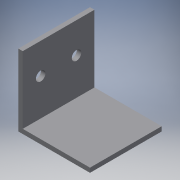
# Autodesk Inventor part: rail gusset
Saved by Autodesk Inventor 2016 (Build 200138000, 138)
## iProperties
Created: 2016-02-08
Part Number: rail gusset
Material: Generic
Document SubType Name: Modeling
Designer: gus
Density: 1 g/cm^3
Appearance: Default
Author: gus
Autodesk Inventor part; units mm, degrees
ref_plane "YZ Plane" through (0, 0, 0) normal (1, 0, 0) x (0, 1, 0)
ref_plane "XZ Plane" through (0, 0, 0) normal (0, 1, 0) x (-1, 0, 0)
ref_plane "XY Plane" through (0, 0, 0) normal (0, 0, 1) x (1, 0, 0)
sketch "Sketch1" plane through (0, 0, 0) normal (0, 0, 1) x (1, 0, 0)
  line L0 (0, 0) -> (47.625, 0)
  line L1 (47.625, 0) -> (47.625, -3.175)
  line L2 (47.625, -3.175) -> (-3.175, -3.175)
  line L3 (-3.175, -3.175) -> (-3.175, 47.625)
  line L4 (-3.175, 47.625) -> (0, 47.625)
  line L5 (0, 47.625) -> (0, 0)
  dimension "d14" = 50.8
  dimension "d15" = 3.175
  constraints: 12 end point, 6 perpendicular, 1 parallel, 1 vertical
  measures "d14" distance of L1.end L2.end
  measures "d15" distance of L0.end L1.end
extrude "Extrusion1" add sketch "Sketch1" along normal blind 50.8
sketch "Sketch2" plane through (0, 0, 0) normal (1, 0, 0) x (0, 0, -1)
  circle A0 centre (-9.525, 22.86) radius 3.3734
  circle A1 centre (-36.5125, 22.86) radius 3.3734
  line L0 (0, 0) -> (-50.8, 0) projected
  line L1 (0, 47.625) -> (0, 0) projected
  line L2 (-50.8, 0) -> (-50.8, 47.625) projected
  dimension "d6" = 6.7469
  dimension "d7" = 6.7469
  dimension "d8" = 22.86
  dimension "d9" = 22.86
  dimension "d16" = 14.2875
  dimension "d17" = 41.275
  constraints: 2 centre point
  measures "d6" diameter of A0
  measures "d7" diameter of A1
  measures "d8" distance from line of L0 A1.centre
  measures "d9" distance from line of L0 A0.centre
  measures "d16" distance from line of L2 A1.centre
  measures "d17" distance from line of L2 A0.centre
extrude "Extrusion2" cut sketch "Sketch2" against normal blind 3.175
sketch "Sketch3" plane through (0, 0, 0) normal (0, 1, 0) x (1, 0, 0)
  line L0 (0, -50.8) -> (-3.175, -50.8) projected
  line L1 (-3.175, -50.8) -> (47.625, -39.0719)
  line L2 (47.625, -50.8) -> (0, -50.8) projected
  circle A0 centre (35.145, -4.1872) radius 3.3734
  circle A1 centre (18.7171, -32.7117) radius 3.3782
  line L3 (-3.175, 0) -> (-3.175, -50.8) projected
  line L4 (-3.175, -50.8) -> (-14.6025, -1.302) construction
  line L5 (47.625, 0) -> (47.625, -50.8) projected
  line L6 (47.625, 0) -> (47.625, -50.8) projected
  line L7 (47.625, -39.0719) -> (47.625, -50.8)
  line L8 (47.625, -50.8) -> (-3.175, -50.8)
  line L9 (-3.175, 0) -> (0, 0) projected
  line L10 (-3.175, 0) -> (47.625, 11.7281)
  line L11 (47.625, 11.7281) -> (47.625, 0)
  line L12 (47.625, 0) -> (-3.175, 0)
  dimension "d18" = 13
  dimension "d19" = 6.7469
  dimension "d20" = 6.7564
  dimension "d21" = 12.7
  dimension "d22" = 50.8
  dimension "d23" = 25.4
  dimension "d24" = 21.8921
  dimension "d25" = 44.45
  dimension "d26" = 12.7
  dimension "d27" = 47.8234
  constraints: 14 end point, 3 collinear, 2 centre point, 1 horizontal, 1 parallel, 1 perpendicular, 1 point on line
  measures "d18" angle of L2 L1
  measures "d19" diameter of A0
  measures "d20" diameter of A1
  measures "d21" distance from line of L1 A1.centre
  measures "d22" distance of L0.end L4.end
  measures "d23" distance from line of L4 A1.centre
  measures "d24" distance from line of L3 A1.centre
  measures "d25" distance edge to line of A0 L4
  measures "d26" distance from line of L10 A0.centre
  measures "d27" distance from line of L4 A0.centre
extrude "Extrusion3" cut sketch "Sketch3" against normal blind 3.175 contours L0 L1 L5 L2 | A0 | A1
extrude "Extrusion4" add sketch "Sketch3" against normal blind 3.175 contours L10 L11 L12 L9
sketch "Sketch4" plane through (0, 0, 0) normal (1, 0, 0) x (0, 0, -1)
  line L0 (-50.8, 0) -> (-50.8, 47.625) projected
  line L1 (0, 47.625) -> (0, 0) projected
  line L2 (-50.8, 47.625) -> (0, 47.625)
  line L3 (0, 47.625) -> (0, 35.56)
  line L4 (0, 35.56) -> (-50.8, 35.56)
  line L5 (-50.8, 35.56) -> (-50.8, 47.625)
  dimension "d32" = 12.065
  constraints: 8 end point, 2 parallel, 1 horizontal, 1 perpendicular, 1 point on line
  measures "d32" distance between parallel lines of L4 L2
extrude "Extrusion5" cut sketch "Sketch4" against normal blind 3.175
body "Solid1"
